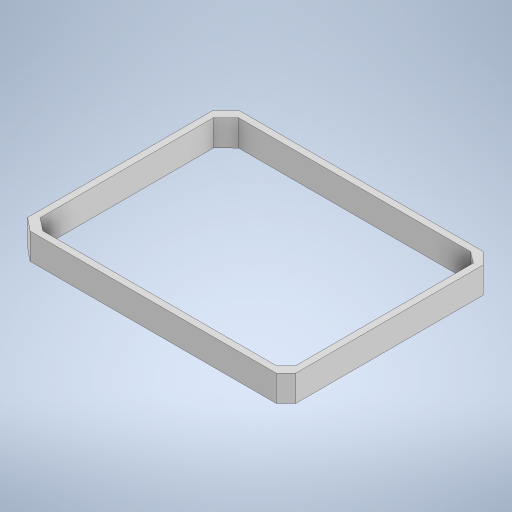
# Autodesk Inventor part: Mash Tank Bottom
Saved by Autodesk Inventor 2024 (Build 280153000, 153)
## iProperties
Created: 2024-11-09
Part Number: Mash Tank Bottom
Material: Generic
Document SubType Name: Modeling
Designer: Emil
Density: 1 g/cm^3
Appearance: Default
Author: Emil
Autodesk Inventor part; units mm, degrees
ref_plane "YZ Plane" through (0, 0, 0) normal (1, 0, 0) x (0, 1, 0)
ref_plane "XZ Plane" through (0, 0, 0) normal (0, 1, 0) x (-1, 0, 0)
ref_plane "XY Plane" through (0, 0, 0) normal (0, 0, 1) x (1, 0, 0)
sketch "Sketch1" plane through (0, 0, 0) normal (0, 1, 0) x (-1, 0, 0)
  line L0 (-35.1948, -29.8974) -> (39.3106, -29.8974)
  line L1 (43.2831, -25.9239) -> (39.3106, -29.8974)
  line L2 (-35.1948, -29.8974) -> (39.3106, -29.8974)
  line L3 (39.3106, -29.8974) -> (43.2831, -25.9239)
  line L4 (43.2831, -25.9239) -> (43.2831, 30.6268)
  line L5 (43.2831, 30.6268) -> (39.3102, 33.8564)
  line L6 (39.3102, 33.8564) -> (-35.8021, 33.8465)
  line L7 (-38.7786, 22.9053) -> (-38.7786, 30.8692)
  line L8 (-35.8021, 33.8465) -> (-38.7786, 30.8692)
  line L9 (-38.7786, 30.8692) -> (-38.7786, -26.3136)
  line L10 (-38.7786, -26.3136) -> (-35.1948, -29.8974)
  line L11 (-35.1948, -29.8974) -> (-38.7786, -26.3136)
  line L12 (-33.3338, -27.8974) -> (37.4464, -27.8974)
  line L13 (41.2831, -24.1074) -> (37.4464, -27.8974)
  line L14 (-33.3338, -27.8974) -> (37.4464, -27.8974)
  line L15 (37.4464, -27.8974) -> (41.2831, -24.1074)
  line L16 (41.2831, -24.1074) -> (41.2831, 28.8221)
  line L17 (41.2831, 28.8221) -> (37.4463, 31.8562)
  line L18 (37.4463, 31.8562) -> (-33.9105, 31.8467)
  line L19 (-36.7786, 21.447) -> (-36.7786, 29.0134)
  line L20 (-33.9105, 31.8467) -> (-36.7786, 29.0134)
  line L21 (-36.7786, 29.0134) -> (-36.7786, -25.3109)
  line L22 (-36.7786, -25.3109) -> (-33.3338, -27.8974)
  line L23 (-33.3338, -27.8974) -> (-36.7786, -25.3109)
  dimension "d1" = 2
  dimension "d2" = 2
  dimension "d3" = 2
  dimension "d4" = 2
  constraints: 48 end point, 6 collinear, 2 horizontal, 2 parallel, 1 vertical
  measures "d1" distance between parallel lines of L18 L6
  measures "d2" distance between parallel lines of L12 L0
  measures "d3" distance between parallel lines of L4 L16
  measures "d4" distance between parallel lines of L21 L9
extrude "Extrusion1" add sketch "Sketch1" along normal blind 8
body "Solid1"
